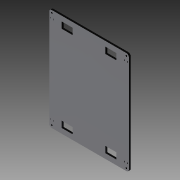
# Autodesk Inventor part: BED PLATE TOP
Saved by Autodesk Inventor 2013 (Build 170138000, 138)
## iProperties
Created: 2014-06-19
Part Number: BED PLATE TOP
Material: Generic
Document SubType Name: Modeling
Designer: employee
Density: 1 g/cm^3
Author: employee
Autodesk Inventor part; units mm, degrees
ref_plane "YZ Plane" through (0, 0, 0) normal (1, 0, 0) x (0, 1, 0)
ref_plane "XZ Plane" through (0, 0, 0) normal (0, 1, 0) x (-1, 0, 0)
ref_plane "XY Plane" through (0, 0, 0) normal (0, 0, 1) x (1, 0, 0)
sketch "Sketch3" plane through (0, 0, 0) normal (0, 0, 1) x (1, 0, 0)
  line L0 (181.0574, -229.1936) -> (181.0574, -225.1936) projected
  line L1 (181.0574, -225.1936) -> (182.5574, -225.1936) projected
  line L2 (182.5574, -225.1936) -> (182.5574, -229.1936) projected
  line L3 (182.5574, -229.1936) -> (181.0574, -229.1936) projected
  line L4 (171.5574, -229.1936) -> (171.5574, -225.1936) projected
  line L5 (171.5574, -225.1936) -> (173.0574, -225.1936) projected
  line L6 (173.0574, -225.1936) -> (173.0574, -229.1936) projected
  line L7 (173.0574, -229.1936) -> (171.5574, -229.1936) projected
  circle A0 centre (179.0574, -242.1936) radius 2.5 projected
  line L8 (112.0574, -234.1936) -> (112.0574, -194.1936) projected
  line L9 (112.0574, -194.1936) -> (147.0574, -194.1936) projected
  line L10 (147.0574, -194.1936) -> (147.0574, -234.1936) projected
  line L11 (147.0574, -234.1936) -> (112.0574, -234.1936) projected
  line L12 (181.0574, 54.8064) -> (181.0574, 50.8064) projected
  line L13 (182.5574, 54.8064) -> (181.0574, 54.8064) projected
  line L14 (182.5574, 50.8064) -> (182.5574, 54.8064) projected
  line L15 (181.0574, 50.8064) -> (182.5574, 50.8064) projected
  line L16 (171.5574, 54.8064) -> (171.5574, 50.8064) projected
  line L17 (173.0574, 54.8064) -> (171.5574, 54.8064) projected
  line L18 (173.0574, 50.8064) -> (173.0574, 54.8064) projected
  line L19 (171.5574, 50.8064) -> (173.0574, 50.8064) projected
  circle A1 centre (179.0574, 67.8064) radius 2.5 projected
  line L20 (112.0574, 59.8064) -> (112.0574, 19.8064) projected
  line L21 (147.0574, 59.8064) -> (112.0574, 59.8064) projected
  line L22 (147.0574, 19.8064) -> (147.0574, 59.8064) projected
  line L23 (112.0574, 19.8064) -> (147.0574, 19.8064) projected
  line L24 (-60.9426, -229.1936) -> (-60.9426, -225.1936) projected
  line L25 (-62.4426, -229.1936) -> (-60.9426, -229.1936) projected
  line L26 (-62.4426, -225.1936) -> (-62.4426, -229.1936) projected
  line L27 (-60.9426, -225.1936) -> (-62.4426, -225.1936) projected
  line L28 (-51.4426, -229.1936) -> (-51.4426, -225.1936) projected
  line L29 (-52.9426, -229.1936) -> (-51.4426, -229.1936) projected
  line L30 (-52.9426, -225.1936) -> (-52.9426, -229.1936) projected
  line L31 (-51.4426, -225.1936) -> (-52.9426, -225.1936) projected
  circle A2 centre (-58.9426, -242.1936) radius 2.5 projected
  line L32 (8.0574, -234.1936) -> (8.0574, -194.1936) projected
  line L33 (-26.9426, -234.1936) -> (8.0574, -234.1936) projected
  line L34 (-26.9426, -194.1936) -> (-26.9426, -234.1936) projected
  line L35 (8.0574, -194.1936) -> (-26.9426, -194.1936) projected
  arc A3 (-66.9426, 49.8064) -> (-64.9426, 47.8064) centre (-64.9426, 49.8064) ccw projected
  line L36 (-64.9426, 47.8064) -> (-58.9426, 47.8064) projected
  line L37 (-58.9426, 47.8064) -> (-58.9426, 57.8064) projected
  line L38 (-58.9426, 57.8064) -> (-54.9426, 57.8064) projected
  line L39 (-54.9426, 57.8064) -> (-54.9426, 47.8064) projected
  line L40 (-54.9426, 47.8064) -> (-48.9426, 47.8064) projected
  arc A4 (-46.9426, 45.8064) -> (-48.9426, 47.8064) centre (-48.9426, 45.8064) ccw projected
  line L41 (-46.9426, 45.8064) -> (-46.9426, -220.1936) projected
  arc A5 (-48.9426, -222.1936) -> (-46.9426, -220.1936) centre (-48.9426, -220.1936) ccw projected
  line L42 (-54.9426, -222.1936) -> (-48.9426, -222.1936) projected
  line L43 (-54.9426, -232.1936) -> (-54.9426, -222.1936) projected
  line L44 (-58.9426, -232.1936) -> (-54.9426, -232.1936) projected
  line L45 (-58.9426, -222.1936) -> (-58.9426, -232.1936) projected
  line L46 (-64.9426, -222.1936) -> (-58.9426, -222.1936) projected
  arc A6 (-64.9426, -222.1936) -> (-66.9426, -224.1936) centre (-64.9426, -224.1936) ccw projected
  line L47 (-66.9426, -242.1936) -> (-66.9426, -224.1936) projected
  arc A7 (-66.9426, -242.1936) -> (-58.9426, -250.1936) centre (-58.9426, -242.1936) ccw projected
  line L48 (179.0574, -250.1936) -> (-58.9426, -250.1936) projected
  arc A8 (179.0574, -250.1936) -> (187.0574, -242.1936) centre (179.0574, -242.1936) ccw projected
  line L49 (187.0574, -242.1936) -> (187.0574, -224.1936) projected
  arc A9 (187.0574, -224.1936) -> (185.0574, -222.1936) centre (185.0574, -224.1936) ccw projected
  line L50 (185.0574, -222.1936) -> (179.0574, -222.1936) projected
  line L51 (179.0574, -222.1936) -> (179.0574, -232.1936) projected
  line L52 (179.0574, -232.1936) -> (175.0574, -232.1936) projected
  line L53 (175.0574, -232.1936) -> (175.0574, -222.1936) projected
  line L54 (175.0574, -222.1936) -> (169.0574, -222.1936) projected
  arc A10 (167.0574, -220.1936) -> (169.0574, -222.1936) centre (169.0574, -220.1936) ccw projected
  line L55 (167.0574, -220.1936) -> (167.0574, 45.8064) projected
  arc A11 (169.0574, 47.8064) -> (167.0574, 45.8064) centre (169.0574, 45.8064) ccw projected
  line L56 (175.0574, 47.8064) -> (169.0574, 47.8064) projected
  line L57 (175.0574, 57.8064) -> (175.0574, 47.8064) projected
  line L58 (179.0574, 57.8064) -> (175.0574, 57.8064) projected
  line L59 (179.0574, 47.8064) -> (179.0574, 57.8064) projected
  line L60 (185.0574, 47.8064) -> (179.0574, 47.8064) projected
  arc A12 (185.0574, 47.8064) -> (187.0574, 49.8064) centre (185.0574, 49.8064) ccw projected
  line L61 (187.0574, 67.8064) -> (187.0574, 49.8064) projected
  arc A13 (187.0574, 67.8064) -> (179.0574, 75.8064) centre (179.0574, 67.8064) ccw projected
  line L62 (-58.9426, 75.8064) -> (179.0574, 75.8064) projected
  arc A14 (-58.9426, 75.8064) -> (-66.9426, 67.8064) centre (-58.9426, 67.8064) ccw projected
  line L63 (-66.9426, 67.8064) -> (-66.9426, 49.8064) projected
  line L64 (8.0574, 59.8064) -> (8.0574, 19.8064) projected
  line L65 (8.0574, 19.8064) -> (-26.9426, 19.8064) projected
  line L66 (-26.9426, 19.8064) -> (-26.9426, 59.8064) projected
  line L67 (-26.9426, 59.8064) -> (8.0574, 59.8064) projected
  circle A15 centre (-58.9426, 67.8064) radius 2.5 projected
  line L68 (-51.4426, 54.8064) -> (-51.4426, 50.8064) projected
  line L69 (-51.4426, 50.8064) -> (-52.9426, 50.8064) projected
  line L70 (-52.9426, 50.8064) -> (-52.9426, 54.8064) projected
  line L71 (-52.9426, 54.8064) -> (-51.4426, 54.8064) projected
  line L72 (-60.9426, 54.8064) -> (-60.9426, 50.8064) projected
  line L73 (-60.9426, 50.8064) -> (-62.4426, 50.8064) projected
  line L74 (-62.4426, 50.8064) -> (-62.4426, 54.8064) projected
  line L75 (-62.4426, 54.8064) -> (-60.9426, 54.8064) projected
  line L76 (-66.9426, 49.8064) -> (-66.9426, -224.1936)
  line L77 (187.0574, -224.1936) -> (187.0574, 49.8064)
  line L78 (-26.9426, 39.8064) -> (8.0574, 39.8064)
  line L79 (112.0574, 39.8064) -> (147.0574, 39.8064)
  line L80 (-26.9426, -214.1936) -> (8.0574, -214.1936)
  line L81 (112.0574, -214.1936) -> (147.0574, -214.1936)
  line L82 (65.0574, 54.8064) -> (65.0574, 30.8064) projected
  arc A16 (65.0574, 30.8064) -> (70.0574, 25.8064) centre (70.0574, 30.8064) ccw projected
  line L83 (70.0574, 25.8064) -> (72.5574, 25.8064) projected
  line L84 (72.5574, 25.8064) -> (72.5574, 13.3064) projected
  arc A17 (47.5574, 13.3064) -> (72.5574, 13.3064) centre (60.0574, 13.3064) ccw projected
  line L85 (47.5574, 13.3064) -> (47.5574, 25.8064) projected
  line L86 (47.5574, 25.8064) -> (50.0574, 25.8064) projected
  arc A18 (50.0574, 25.8064) -> (55.0574, 30.8064) centre (50.0574, 30.8064) ccw projected
  line L87 (55.0574, 30.8064) -> (55.0574, 54.8064) projected
  arc A19 (65.0574, 54.8064) -> (55.0574, 54.8064) centre (60.0574, 54.8064) ccw projected
  point P0 (0, 0)
  constraints: 12 end point, 8 midpoint, 4 tangent, 1 collinear, 1 parallel, 1 perpendicular
extrude "Extrusion3" add sketch "Sketch3" along normal blind 5.715 contours L8 L9 L10 L81 | L79 L22 L23 L20 | L80 L34 L35 L32 | L63 A14 L62 A13 L61 A12 L60 L59 L58 L57 L56 A11 L55 A10 L54 L53 L52 L51 L50 A9 L49 A8 L48 A7 L47 A6 L46 L45 L44 L43 L42 A5 L41 A4 L40 L39 L38 L37 L36 A3 | A3 L36 L37 L38 L39 L40 A4 L41 A5 L42 L43 L44 L45 L46 A6 L76 | L77 A9 L50 L51 L52 L53 L54 A10 L55 A11 L56 L57 L58 L59 L60 A12 | L64 L65 L66 L78 | L82 A16 L83 L84 A17 L85 L86 A18 L87 A19
sketch "Sketch4" plane through (0, 0, 5.715) normal (0, 0, 1) x (1, 0, 0)
  line L0 (187.0574, -242.1936) -> (187.0574, 67.8064) projected
  line L1 (179.0574, 75.8064) -> (-58.9426, 75.8064) projected
  line L2 (-52.9426, 25.8064) -> (173.0574, 25.8064)
  line L3 (173.0574, 25.8064) -> (173.0574, -200.1936)
  line L4 (173.0574, -200.1936) -> (-52.9426, -200.1936)
  line L5 (-52.9426, -200.1936) -> (-52.9426, 25.8064)
  point P0 (0, 0)
  point P1 (60.0574, 25.8064)
  point P2 (60.0574, 75.8064)
  point P3 (173.0574, -87.1936)
  point P4 (187.0574, -87.1936)
  dimension "d8" = 226
  constraints: 8 end point, 4 midpoint, 2 parallel, 2 perpendicular, 1 horizontal, 1 horizontal alignment, 1 vertical alignment
  measures "d8" distance of L2.end L3.end
extrude "Extrusion4" cut sketch "Sketch4" against normal through all
sketch "Sketch5" plane through (0, 0, 5.715) normal (0, 0, 1) x (1, 0, 0)
  line L0 (-52.9426, 25.8064) -> (173.0574, 25.8064) projected
  line L1 (147.0574, 39.8064) -> (112.0574, 39.8064) projected
  line L2 (179.0574, 75.8064) -> (-58.9426, 75.8064) projected
  line L3 (55.0574, 25.8064) -> (55.0574, 59.8064)
  line L4 (55.0574, 59.8064) -> (65.0574, 59.8064)
  line L5 (65.0574, 59.8064) -> (65.0574, 25.8064)
  point P0 (0, 0)
  point P1 (60.0574, 59.8064)
  point P2 (60.0574, 25.8064)
  dimension "d12" = 10
  dimension "d15" = 20
  constraints: 6 end point, 3 perpendicular, 2 midpoint, 2 point on line, 1 vertical alignment
  measures "d12" distance of L3.end L4.end
  measures "d15" distance between parallel lines of L4 L1
extrude "Extrusion5" cut sketch "Sketch5" against normal through all
fillet "Fillet1" radius 5 4 edges at (55.0574, 25.8064, 2.8575) (55.0574, 59.8064, 2.8575) (65.0574, 59.8064, 2.8575) (65.0574, 25.8064, 2.8575)
body "Solid2"
